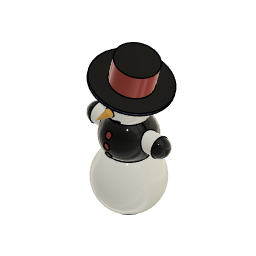
P10 (Autodesk Fusion 360 design; units mm, degrees)
Autodesk Fusion 360 part; units mm, degrees
sketch "Sketch1" plane through (0, 0, 0) normal (0, 1, 0) x (1, 0, 0)
  line L0 (0, 0) -> (0, -225) construction
  line L1 (0, 0) -> (108.9725, 0)
  line L2 (0, -225) -> (0, -475) construction
  arc A0 (0, -475) -> (108.9725, 0) centre (0, -225) ccw
  line L3 (0, -475) -> (0, 0)
  dimension "d1" = 225
  dimension "d2" = 500
  constraint coincident L0.start L1.start
  constraint vertical L0
  constraint coincident L0.end L2.start
  constraint perpendicular L0 L1
  constraint parallel L0 L2
  measures "d1" distance of L0.start L0.end
  measures "d2" diameter of A0
revolve "Revolve1" add sketch "Sketch1" angle 360 about axis through (0, 0, 0) along (0, 0, 1)
sketch "Sketch2" plane through (0, 0, 0) normal (0, 1, 0) x (1, 0, 0)
  line L0 (0, 0) -> (0, -550) construction
  line L1 (0, -375) -> (0, -725)
  ellipse E0 centre (0, -550) end of major axis (200, -550) minor radius 175 (0, -725) -> (0, -375) ccw
  dimension "d4" = 550
  dimension "d5" = 400
  dimension "d6" = 350
  constraint coincident L0.start origin
  constraint vertical L0
  constraint coincident L0.end E0.centre
  constraint vertical L1
  measures "d4" distance of L0.start L0.end
  measures "d5" distance of E0
revolve "Revolve2" add sketch "Sketch2" angle 360 about axis through (0, 0, 0) along (0, 0, 1)
sketch "Sketch3" plane through (0, 0, 0) normal (0, 1, 0) x (1, 0, 0)
  line L0 (0, 0) -> (0, -825) construction
  line L1 (0, -1000) -> (0, -650)
  arc A0 (0, -1000) -> (0, -650) centre (0, -825) ccw
  dimension "d8" = 825
  dimension "d9" = 350
  constraint coincident L0.start origin
  constraint vertical L0
  constraint coincident L0.end A0.centre
  constraint coincident L0 L1.end
  constraint parallel L0 L1
  measures "d8" distance of L0.start L0.end
  measures "d9" diameter of A0
revolve "Revolve3" add sketch "Sketch3" angle 360 about axis through (0, 0, 0) along (0, 0, 1)
sketch "Sketch4" plane through (0, 0, 0) normal (0, 1, 0) x (1, 0, 0)
  line L0 (0, 0) -> (0, -580) construction
  line L1 (0, -580) -> (550, -580) construction
  line L2 (0, -580) -> (275, -580)
  line L3 (275, -580) -> (350, -580)
  arc A0 (275, -655) -> (350, -580) centre (275, -580) ccw
  line L4 (275, -655) -> (0, -655)
  line L5 (0, -655) -> (0, -580)
  dimension "d11" = 580
  dimension "d12" = 275
  dimension "d13" = 150
  constraint coincident L0.start origin
  constraint vertical L0
  constraint perpendicular L0 L1
  constraint perpendicular L0 L2
  constraint coincident L2.end L3.start
  constraint coincident L1 L3.end
  constraint horizontal L4
  constraint perpendicular L2 L5
  constraint tangent A0 L4
  measures "d11" distance of L0.start L0.end
  measures "d12" distance of L0.end L2.end
  measures "d13" diameter of A0
revolve "Revolve4" add sketch "Sketch4" angle 360 about axis through (275, 0, 580) along (1, 0, 0)
mirror "Mirror1" about plane through (0, 0, 0) normal (1, 0, 0) of "Revolve4"
ref_plane "WorkPlane1" through (0, -205, 0) normal (0, 1, 0) x (0, 0, 1)
sketch "Sketch5" plane through (0, -205, 0) normal (0, 1, 0) x (1, 0, 0)
  line L0 (0, 0) -> (0, -475) construction
  line L1 (0, 0) -> (0, -550) construction
  line L2 (0, 0) -> (0, -625) construction
  circle A0 centre (0, -550) radius 25
  circle A1 centre (0, -625) radius 25
  circle A2 centre (0, -475) radius 25
  dimension "d18" = 475
  dimension "d19" = 550
  dimension "d20" = 625
  dimension "d23" = 50
  dimension "d24" = 50
  dimension "d25" = 50
  constraint coincident L0.start L1.start
  constraint vertical L0
  constraint parallel L0 L1
  constraint parallel L0 L2
  constraint coincident L1.end A0.centre
  constraint coincident L2.end A1.centre
  constraint coincident L0.end A2.centre
  measures "d18" distance of L0.start L0.end
  measures "d19" distance of L0.start L1.end
  measures "d20" distance of L0.start L2.end
  measures "d23" diameter of A0
  measures "d24" diameter of A1
  measures "d25" diameter of A2
extrude "Extrude1" add sketch "Sketch5" along normal up to surface end surface at (162.2203, -75.3402, 471.6964)
sketch "Sketch6" plane through (0, 0, 0) normal (1, 0, 0) x (0, 1, 0)
  line L0 (0, 0) -> (0, 550) construction
  line L1 (-300, 662.5) -> (-300, 437.5)
  line L2 (-300, 662.5) -> (-160, 662.5)
  line L3 (-300, 437.5) -> (-160, 437.5)
  arc A0 (-160, 662.5) -> (-160, 437.5) centre (-29.9069, 550) ccw
  dimension "d28" = 550
  dimension "d31" = 225
  dimension "d32" = 140
  dimension "d33" = 140
  constraint coincident L0.start origin
  constraint vertical L0
  constraint perpendicular L1 L2
  constraint perpendicular L1 L3
  measures "d28" distance of L0.start L0.end
  measures "d31" distance of L1.start L1.end
  measures "d32" distance of L1.start L2.end
  measures "d33" distance of L1.end L3.end
revolve "Revolve5" cut sketch "Sketch6" angle 45 about axis through (0, 0, 0) along (0, 0, 1) second angle 45
sketch "Sketch7" plane through (0, -205, 0) normal (0, 1, 0) x (1, 0, 0)
  line L0 (0, 0) -> (0, -25) construction
  line L1 (0, -25) -> (0, -1000) construction
  line L2 (0, 0) -> (0, -840)
  line L3 (0, -690) -> (90, -690) construction
  arc A0 (87.5, -757.8797) -> (-87.5, -757.8797) centre (0, -840) ccw construction
  circle A1 centre (15, -720.9412) radius 12.5
  circle A2 centre (45, -728.757) radius 12.5
  circle A3 centre (-15, -720.9412) radius 12.5
  circle A4 centre (-45, -728.757) radius 12.5
  line L4 (0, 0) -> (0, -875) construction
  line L5 (0, -875) -> (70, -875) construction
  circle A5 centre (70, -875) radius 32.5
  line L6 (0, -875) -> (-70, -875) construction
  circle A6 centre (-70, -875) radius 32.5
  dimension "d36" = 840
  dimension "d37" = 240
  dimension "d40" = 175
  dimension "d41" = 25
  dimension "d42" = 25
  dimension "d43" = 25
  dimension "d44" = 25
  dimension "d45" = 15
  dimension "d46" = 30
  dimension "d47" = 15
  dimension "d48" = 30
  dimension "d49" = 875
  dimension "d50" = 70
  dimension "d51" = 65
  dimension "d52" = 70
  dimension "d53" = 65
  constraint coincident L0.start L2.start
  constraint vertical L0
  constraint parallel L0 L1
  constraint parallel L1 L2
  constraint coincident L2.end A0.centre
  constraint coincident L2 L3.start
  constraint perpendicular L1 L3
  constraint coincident A0 A1.centre
  constraint coincident A0 A2.centre
  constraint coincident A0 A3.centre
  constraint coincident A0 A4.centre
  constraint parallel L1 L4
  constraint perpendicular L4 L5
  constraint coincident L5.end A5.centre
  constraint perpendicular L4 L6
  constraint coincident L6.end A6.centre
  measures "d36" distance of L0.start L2.end
  measures "d37" diameter of A0
  measures "d40" distance of A0.start A0.end
  measures "d41" diameter of A1
  measures "d42" diameter of A2
  measures "d43" diameter of A3
  measures "d44" diameter of A4
  measures "d45" distance of L2 A1.centre
  measures "d46" horizontal distance of A1.centre A2.centre
  measures "d47" distance of L1 A3.centre
  measures "d48" horizontal distance of A3.centre A4.centre
  measures "d49" distance of L0.start L4.end
  measures "d50" distance of L4.end L5.end
  measures "d51" diameter of A5
  measures "d52" distance of L4.end L6.end
  measures "d53" diameter of A6
extrude "Extrude2" add sketch "Sketch7" along normal blind 100
sketch "Sketch8" plane through (0, 0, 0) normal (1, 0, 0) x (0, 1, 0)
  line L0 (0, 1000) -> (0, 700)
  line L1 (0, 700) -> (-270, 700)
  line L2 (-270, 700) -> (-270, 1000)
  line L3 (-270, 1000) -> (0, 1000)
  arc A0 (-53.3876, 1000) -> (-130, 700) centre (11.4796, 823.6521) ccw
  dimension "d56" = 300
  dimension "d57" = 270
  constraint vertical L0
  constraint perpendicular L0 L1
  constraint perpendicular L1 L2
  constraint perpendicular L0 L3
  constraint coincident L3 A0.start
  constraint coincident L1 A0.end
  measures "d56" distance of L0.start L0.end
  measures "d57" distance of L0.end L1.end
revolve "Revolve6" cut sketch "Sketch8" angle 45 about axis through (0, 0, 1000) along (0, 0, -1) second angle 45 contours L1 L2 L3 A0
sketch "Sketch9" plane through (0, 0, 0) normal (1, 0, 0) x (0, 1, 0)
  line L0 (0, 0) -> (0, 800) construction
  line L1 (0, 800) -> (-300, 800)
  line L2 (0, 725) -> (0, 880.3848)
  line L3 (-300, 800) -> (0, 880.3848)
  dimension "d60" = 800
  dimension "d61" = 300
  dimension "d62" = 15
  constraint coincident L0.start origin
  constraint vertical L0
  constraint perpendicular L0 L1
  constraint coincident L0 L2.start
  constraint perpendicular L1 L2
  measures "d60" distance of L0.start L0.end
  measures "d61" distance of L0.end L1.end
  measures "d62" angle of L1 L3
revolve "Revolve7" add sketch "Sketch9" angle 360 about axis through (0, 0, 800) along (0, -1, 0) second angle 360
sketch "Sketch10" plane through (0, 0, 0) normal (0, 1, 0) x (1, 0, 0)
  line L0 (0, 0) -> (0, -875) construction
  line L1 (0, 0) -> (0, -875) construction
  line L2 (0, -875) -> (111.4453, -1290.9194) construction
  line L3 (0, -875) -> (0, -1297) construction
  line L4 (28.4701, -981.2518) -> (138.4701, -951.7774)
  line L5 (138.4701, -951.7774) -> (130.7055, -922.7997)
  line L6 (130.7055, -922.7997) -> (294.8811, -878.8089)
  line L7 (294.8811, -878.8089) -> (300.0575, -898.1274)
  line L8 (300.0575, -898.1274) -> (175.6004, -931.4756)
  line L9 (175.6004, -931.4756) -> (224.776, -1115.0015)
  line L10 (224.776, -1115.0015) -> (75.0575, -1155.1185)
  line L11 (28.4701, -981.2518) -> (75.0575, -1155.1185)
  dimension "d66" = 875
  dimension "d67" = 15
  dimension "d68" = 110
  dimension "d69" = 30
  dimension "d70" = 110
  dimension "d74" = 210
  dimension "d75" = 155
  dimension "d76" = 190
  dimension "d77" = 225
  dimension "d78" = 422
  constraint coincident L0.start L1.start
  constraint vertical L0
  constraint parallel L0 L1
  constraint vertical L3
  constraint coincident L2 L4.start
  constraint perpendicular L2 L4
  constraint perpendicular L4 L5
  constraint perpendicular L5 L6
  constraint perpendicular L4 L7
  constraint perpendicular L7 L8
  constraint perpendicular L8 L9
  constraint coincident L2 L10.end
  constraint perpendicular L2 L10
  constraint coincident L0.end L1.end
  measures "d66" distance of L0.start L0.end
  measures "d67" angle of L2 L3
  measures "d68" distance of L0.end L4
  measures "d69" distance of L4.end L5.end
  measures "d70" horizontal distance of L4.start L4.end
  measures "d74" distance of L6 L10
  measures "d75" distance of L9.end L10.end
  measures "d76" distance of L8 L10
  measures "d77" horizontal distance of L7.end L10.end
  measures "d78" distance of L0.end L3.end
revolve "Revolve8" add sketch "Sketch10" angle 360 about axis through (28.4701, 0, 981.2518) along (0.258819, 0, 0.965926) second angle 360
